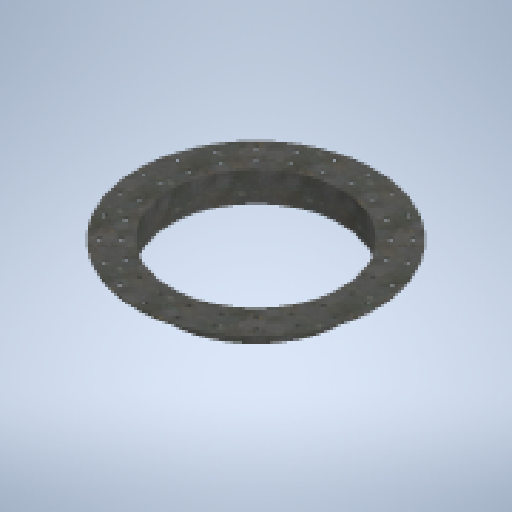
# Autodesk Inventor part: Brida_cuello_tapa
Saved by Autodesk Inventor 2023 (Build 270158000, 158)
## iProperties
Created: 2022-11-02
Part Number: Brida_cuello_tapa
Material: Steel ASTM A36
Document SubType Name: Modeling
Designer: Juanse
Density: 7.85 g/cm^3
Appearance: Plate
Mass: 21448 g
Surface Area: 9507.77 cm^2
Volume: 2732.23 cm^3
Part_Area: 95077.668
Author: Juanse
Autodesk Inventor part; units mm, degrees
ref_plane "YZ Plane" through (0, 0, 0) normal (1, 0, 0) x (0, 1, 0)
ref_plane "XZ Plane" through (0, 0, 0) normal (0, 1, 0) x (-1, 0, 0)
ref_plane "XY Plane" through (0, 0, 0) normal (0, 0, 1) x (1, 0, 0)
sketch "Sketch1" plane through (0, 0, 0) normal (0, 0, 1) x (1, 0, 0)
  line L0 (-299, -106) -> (-299, 0)
  line L1 (-299, 0) -> (-420, 0)
  line L2 (-420, 0) -> (-420, -6)
  line L3 (-420, -6) -> (-305, -6)
  line L4 (-305, -6) -> (-305, -106)
  line L5 (-305, -106) -> (-299, -106)
  line L6 (0, 0) -> (0, -106)
  dimension "d0" = 6
  dimension "d1" = 6
  dimension "d2" = 610
  dimension "d3" = 840
  dimension "d4" = 100
  constraints: 14 end point, 4 perpendicular, 2 horizontal alignment, 2 vertical, 1 parallel
  measures "d0" distance between parallel lines of L0 L4
  measures "d1" distance between parallel lines of L1 L3
  measures "d2" diameter of L4 L6
  measures "d3" diameter of L2 L6
  measures "d4" distance of L3.end L4.end
revolve "Revolution1" add sketch "Sketch1" angle 360 about axis through (0, 0, 0) along (0, -1, 0)
sketch "Sketch2" plane through (0, 0, 0) normal (0, 1, 0) x (1, 0, 0)
  circle A0 centre (-335, 0) radius 7.1437
  circle A1 centre (-390, 0) radius 7.1437
  circle A2 centre (0, 0) radius 335 construction
  circle A3 centre (0, 0) radius 390 construction
  dimension "d9" = 670
  dimension "d10" = 780
  dimension "d6" = 14.2875
  dimension "d7" = 14.2875
  constraints: 4 horizontal alignment, 2 centre point, 2 coincident, 4 other
  measures "d6" diameter of A0
  measures "d7" diameter of A1
extrude "Extrusion1" cut sketch "Sketch2" against normal through all
pattern_circular "Circular Pattern1" count 24 over 360 about axis through (0, -53, 0) along (0, 1, 0) of "Extrusion1"
equation "\"d1\" = d0"
equation "\"d7\" = d6"
equation "\"Part_Area\" = 95077.667828"
body "Solid1"
